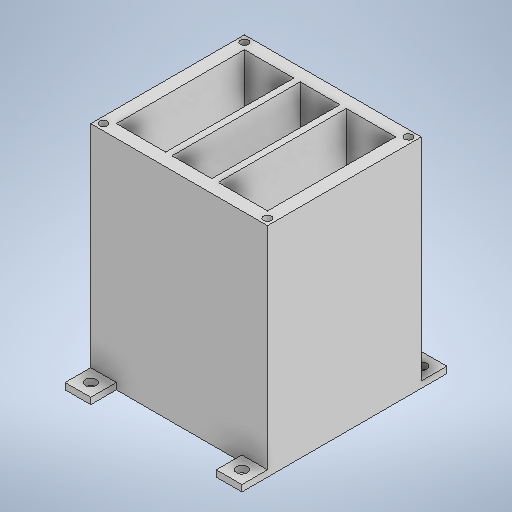
# Autodesk Inventor part: switch_pannel_box
Saved by Autodesk Inventor 2025 (Build 290162000, 162)
## iProperties
Created: 2025-01-22
Part Number: switch_pannel_box
Material: Generic
Document SubType Name: Modeling
Designer: danielrachi
Density: 1 g/cm^3
Appearance: Default
Author: danielrachi
Autodesk Inventor part; units mm, degrees
ref_plane "YZ Plane" through (0, 0, 0) normal (1, 0, 0) x (0, 1, 0)
sketch "Sketch1" plane through (0, 0, 0) normal (0, 1, 0) x (-1, 0, 0)
  point P0 (0, 0)
sketch "Sketch2" plane through (0, 0, 0) normal (0, 1, 0) x (-1, 0, 0)
  line L0 (34.5, 30) -> (-34.5, 30)
  line L1 (-34.5, 30) -> (-34.5, -30)
  line L2 (-34.5, -30) -> (34.5, -30)
  line L3 (34.5, -30) -> (34.5, 30)
  line L4 (34.5, 30) -> (-34.5, -30) construction
  line L5 (-34.5, 30) -> (34.5, -30) construction
  point P0 (0, 0)
  dimension "d0" = 69
  dimension "d1" = 60
  constraints: 12 end point, 2 midpoint, 2 parallel, 1 horizontal, 1 perpendicular
  measures "d0" distance of L2.end L1.end
  measures "d1" distance of L1.end L0.end
extrude "Extrusion1" add sketch "Sketch2" along normal blind 85
sketch "Sketch3" plane through (0, 85, 0) normal (0, 1, 0) x (1, 0, 0)
  line L0 (-29.5, -25) -> (29.5, -25)
  line L1 (29.5, -25) -> (29.5, 25)
  line L2 (29.5, 25) -> (-29.5, 25)
  line L3 (-29.5, 25) -> (-29.5, -25)
  line L4 (-29.5, -25) -> (29.5, 25) construction
  line L5 (29.5, -25) -> (-29.5, 25) construction
  point P0 (0, 0)
  dimension "d4" = 59
  dimension "d5" = 50
  constraints: 12 end point, 2 midpoint, 2 parallel, 1 horizontal, 1 perpendicular
  measures "d4" distance of L2.end L1.end
  measures "d5" distance of L1.end L0.end
extrude "Extrusion2" cut sketch "Sketch3" against normal blind 80
sketch "Sketch4" plane through (0, 85, 0) normal (0, 1, 0) x (1, 0, 0)
  circle A0 centre (32, -27.5) radius 1.55
  line L0 (-34.5, -30) -> (34.5, -30) projected
  line L1 (34.5, -30) -> (34.5, 30) projected
  circle A1 centre (32, 27.5) radius 1.55
  circle A2 centre (-32, 27.5) radius 1.55
  circle A3 centre (-32, -27.5) radius 1.55
  line L2 (34.5, 30) -> (-34.5, 30) projected
  line L3 (-34.5, 30) -> (-34.5, -30) projected
  point P0 (0, 0)
  dimension "d8" = 3.1
  dimension "d9" = 2.5
  dimension "d10" = 2.5
  dimension "d11" = 2.5
  dimension "d12" = 2.5
  constraints: 4 centre point, 3 equal radius, 2 horizontal alignment, 2 vertical alignment
  measures "d8" diameter of A0
  measures "d9" distance from line of A0.centre L0
  measures "d10" distance from line of A0.centre L1
  measures "d11" distance from line of A2.centre L2
  measures "d12" distance from line of L3 A2.centre
extrude "Extrusion3" cut sketch "Sketch4" against normal blind 10 contours A0 | A1 | A2 | A3
sketch "Sketch5" plane through (-34.5, 0, 30) normal (0, 0, 1) x (1, 0, 0)
  line L0 (0, 0) -> (0, 85) projected
  line L1 (0, 0) -> (10, 0)
  line L2 (10, 0) -> (10, 2.5)
  line L3 (10, 2.5) -> (0, 2.5)
  line L4 (0, 2.5) -> (0, 0)
  line L5 (34.5, 0) -> (34.5, 85)
  line L6 (5, 85) -> (64, 85) projected
  line L7 (69, 0) -> (59, 0)
  line L8 (59, 0) -> (59, 2.5)
  line L9 (59, 2.5) -> (69, 2.5)
  line L10 (69, 2.5) -> (69, 0)
  dimension "d15" = 10
  dimension "d16" = 2.5
  constraints: 18 end point, 4 symmetric about line, 2 parallel, 1 horizontal, 1 midpoint, 1 perpendicular
  measures "d15" distance of L3.end L2.end
  measures "d16" distance of L2.end L1.end
extrude "Extrusion4" add sketch "Sketch5" along normal blind 10
sketch "Sketch6" plane through (-34.5, 2.5, 30) normal (0, 1, 0) x (1, 0, 0)
  circle A0 centre (5, -5) radius 2.1
  line L0 (10, -10) -> (0, -10) projected
  line L1 (0, 0) -> (0, -10) projected
  line L2 (69, 60) -> (0, 60) projected
  line L3 (34.5, 60) -> (34.5, 0)
  line L4 (0, 0) -> (69, 0) projected
  circle A1 centre (64, -5) radius 2.1
  point P0 (34.5, 30)
  dimension "d19" = 4.2
  dimension "d20" = 5
  dimension "d21" = 5
  constraints: 2 centre point, 2 end point, 2 midpoint, 1 symmetric about line, 1 other
  measures "d19" diameter of A0
  measures "d20" distance from line of A0.centre L0
  measures "d21" distance from line of A0.centre L1
extrude "Extrusion5" cut sketch "Sketch6" against normal up to next
ref_plane "Work Plane2" through (-34.5, 85, 0) normal (0, 0, 1) x (1, 0, 0)
mirror "Mirror2" about plane through (-34.5, 85, 0) normal (0, 0, 1) of "Extrusion4", "Extrusion5"
sketch "Sketch7" plane through (34.5, 85, -30) normal (0, 0, -1) x (-1, 0, 0)
  line L0 (5, 0) -> (5, -80) projected
  line L1 (64, 0) -> (64, -80) projected
  line L2 (5, -80) -> (64, -80)
  line L3 (64, -80) -> (64, -50)
  line L4 (64, -50) -> (5, -50)
  line L5 (5, -50) -> (5, -80)
  point P0 (34.5, -85)
  point P1 (5, -50)
  dimension "d24" = 30
  constraints: 8 end point, 2 parallel, 1 horizontal, 1 perpendicular, 1 point on line
  measures "d24" distance of L3.end L2.end
extrude "Extrusion6" cut sketch "Sketch7" against normal up to next
sketch "Sketch8" plane through (0, 5, 0) normal (0, 1, 0) x (1, 0, 0)
  line L0 (-29.5, 25) -> (29.5, 25) projected
  line L1 (-6.5, -25) -> (6.5, -25)
  line L2 (6.5, -25) -> (6.5, 25)
  line L3 (6.5, 25) -> (-6.5, 25)
  line L4 (-6.5, 25) -> (-6.5, -25)
  line L5 (-6.5, -25) -> (6.5, 25) construction
  line L6 (6.5, -25) -> (-6.5, 25) construction
  line L7 (29.5, -25) -> (-29.5, -25) projected
  line L8 (-6.5, 25) -> (-11.5, 25)
  line L9 (-11.5, 25) -> (-11.5, -25)
  line L10 (-11.5, -25) -> (-6.5, -25)
  line L11 (-6.5, -25) -> (-6.5, 25)
  line L12 (6.5, -25) -> (11.5, -25)
  line L13 (11.5, -25) -> (11.5, 25)
  line L14 (11.5, 25) -> (6.5, 25)
  line L15 (6.5, 25) -> (6.5, -25)
  line L16 (-10.25, 25) -> (-7.75, 25)
  line L17 (-7.75, 25) -> (-7.75, -26.1279)
  line L18 (-7.75, -26.1279) -> (-10.25, -26.1279)
  line L19 (-10.25, -26.1279) -> (-10.25, 25)
  point P0 (0, 0)
  point P1 (-10.25, -25)
  point P2 (-7.75, -25)
  dimension "d27" = 13
  dimension "d28" = 5
  dimension "d29" = 5
  dimension "d30" = 1.25
  dimension "d31" = 1.25
  constraints: 36 end point, 8 parallel, 4 horizontal, 4 perpendicular, 4 point on line, 2 midpoint
  measures "d27" distance of L3.end L2.end
  measures "d28" distance of L10.end L9.end
  measures "d29" distance of L14.end L13.end
  measures "d30" distance between parallel lines of L19 L9
  measures "d31" distance between parallel lines of L17 L4
extrude "Extrusion7" add sketch "Sketch8" along normal blind 80 contours L0 L17 L7 L19
ref_plane "Work Plane3" through (0, 85, 25) normal (1, 0, 0) x (0, 0, -1)
mirror "Mirror3" about plane through (0, 85, 25) normal (1, 0, 0) of "Extrusion7"
sketch "Sketch9" plane through (10.25, 35, -25) normal (0, 0, -1) x (-1, 0, 0)
  line L0 (0, -30) -> (0, 50) projected
  line L1 (2.5, 0) -> (2.5, 50) projected
  line L2 (0, -30) -> (2.5, -30)
  line L3 (2.5, -30) -> (2.5, 0)
  line L4 (2.5, 0) -> (0, 0)
  line L5 (0, 0) -> (0, -30)
  line L6 (18, -30) -> (18, 0) projected
  line L7 (20.5, 50) -> (20.5, -30) projected
  line L8 (18, -30) -> (20.5, -30)
  line L9 (20.5, -30) -> (20.5, 0)
  line L10 (20.5, 0) -> (18, 0)
  line L11 (18, 0) -> (18, -30)
  point P0 (10.25, -35)
  constraints: 16 end point, 4 parallel, 2 horizontal, 2 perpendicular, 2 point on line
extrude "Extrusion8" add sketch "Sketch9" along normal blind 5
equation "\"d0\" = external_len"
equation "\"d1\" = external_width"
equation "\"d2\" = internal_height + thickness"
equation "\"d4\" = internal_len"
equation "\"d5\" = internal_width"
equation "\"d6\" = internal_height"
equation "\"d32\" = internal_height"
equation "\"d34\" = thickness"
equation "\"external_len\" = 69"
equation "\"external_width\" = 60"
equation "\"thickness\" = 5"
equation "\"internal_height\" = 80"
equation "\"separator_thickness\" = 2.5"
equation "\"switch_len_at_clip\" = 13"
equation "\"internal_len\" = external_len - 2 * thickness"
equation "\"internal_width\" = external_width - 2 * thickness"
body "Solid1"
